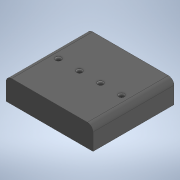
# Autodesk Inventor part: 4aa-holder
Saved by Autodesk Inventor 2020 (Build 240168000, 168)
## iProperties
Created: 2020-11-03
Part Number: 4aa-holder
Material: Generic
Document SubType Name: Modeling
Designer: alnwlsn
Density: 1 g/cm^3
Appearance: Default
Author: alnwlsn
Autodesk Inventor part; units mm, degrees
ref_plane "YZ Plane" through (0, 0, 0) normal (1, 0, 0) x (0, 1, 0)
ref_plane "XZ Plane" through (0, 0, 0) normal (0, 1, 0) x (-1, 0, 0)
ref_plane "XY Plane" through (0, 0, 0) normal (0, 0, 1) x (1, 0, 0)
sketch "Sketch1" plane through (0, 0, 0) normal (0, 0, 1) x (1, 0, 0)
  line L0 (0, 0) -> (62, 0)
  line L1 (62, 0) -> (62, 12)
  line L2 (58, 16) -> (4, 16)
  line L3 (0, 12) -> (0, 0)
  arc A0 (4, 16) -> (0, 12) centre (4, 12) ccw
  arc A1 (62, 12) -> (58, 16) centre (58, 12) ccw
  point P0 (0, 16)
  dimension "d0" = 16
  dimension "d1" = 62
  dimension "d2" = 4
  constraints: 8 end point, 4 point on circle, 4 tangent, 2 centre point, 2 parallel, 2 point on line, 1 equal radius, 1 horizontal, 1 perpendicular
  measures "d0" distance of point (0, 16) L0.start
  measures "d1" distance of L0.start L0.end
  measures "d2" radius of A0
extrude "Extrusion1" add sketch "Sketch1" along normal blind 57.7
sketch "Sketch2" plane through (0, 0, 0) normal (0, -1, 0) x (1, 0, 0)
  line L0 (62, 0) -> (62, 57.7) projected
  line L1 (62, 28.85) -> (0, 28.85) construction
  line L2 (0, 0) -> (0, 57.7) projected
  circle A0 centre (31, 28.85) radius 22.5 construction
  circle A1 centre (53.5, 28.85) radius 2
  circle A2 centre (8.5, 28.85) radius 2
  circle A3 centre (31, 28.85) radius 7.5 construction
  circle A4 centre (38.5, 28.85) radius 2
  circle A5 centre (23.5, 28.85) radius 2
  dimension "d5" = 45
  dimension "d8" = 4
  dimension "d9" = 15
  constraints: 6 centre point, 4 point on circle, 4 point on line, 3 equal radius, 3 midpoint, 2 end point, 1 coincident
  measures "d5" diameter of A0
  measures "d8" diameter of A1
  measures "d9" diameter of A3
extrude "Extrusion2" cut sketch "Sketch2" against normal through all
body "Solid1"
